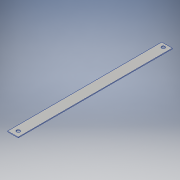
# Autodesk Inventor part: support_lateral
Saved by Autodesk Inventor 2019 (Build 230136000, 136)
## iProperties
Created: 2019-03-26
Part Number: support_lateral
Material: Aluminium 6061
Document SubType Name: Modeling
Designer: theor
Density: 2.7 g/cm^3
Appearance: Aluminium - Plat
Author: theor
Autodesk Inventor part; units mm, degrees
ref_plane "YZ Plane" through (0, 0, 0) normal (1, 0, 0) x (0, 1, 0)
ref_plane "XZ Plane" through (0, 0, 0) normal (0, 1, 0) x (-1, 0, 0)
ref_plane "XY Plane" through (0, 0, 0) normal (0, 0, 1) x (1, 0, 0)
sketch "Esquisse2" plane through (0, 0, 0) normal (0, 1, 0) x (-1, 0, 0)
  line L0 (-7, 103) -> (7, 103)
  line L1 (7, 103) -> (7, -103)
  line L2 (7, -103) -> (-7, -103)
  line L3 (-7, -103) -> (-7, 103)
  line L4 (-7, 103) -> (7, -103) construction
  line L5 (7, 103) -> (-7, -103) construction
  point P0 (0, 0)
  dimension "d0" = 206
  dimension "d1" = 14
  constraints: 12 end point, 2 midpoint, 2 parallel, 1 horizontal, 1 perpendicular
  measures "d0" distance of L2.end L0.start
  measures "d1" distance of L1.end L2.end
extrude "Extrusion1" add sketch "Esquisse2" along normal blind 1
sketch "Esquisse3" plane through (0, 1, 0) normal (0, 1, 0) x (1, 0, 0)
  line L0 (7, 103) -> (-7, 103) projected
  line L1 (-7, -103) -> (7, -103) projected
  point P0 (0, 0)
  point P1 (0, -96)
  point P2 (0, 98)
  dimension "d4" = 5
  dimension "d14" = 194
  constraints: 2 vertical alignment
  measures "d4" distance from line of point (0, 98) L0
  measures "d14" distance of point (0, 98) point (0, -96)
hole "Perçage1" at (0, 1, 96) at (0, 1, -98) direction (0, -1, 0) diameter 4.5 end through all clearance for "Vis d'assemblage à six pans creux ISO 4762" size "M4" standard "ISO"
